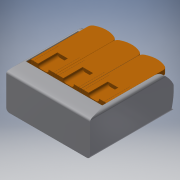
# Autodesk Inventor part: fc17-134
Saved by Autodesk Inventor 2017.1 (Build 211199000, 199)
## iProperties
Category: Electrical
Company: Autodesk Inc.
Created: 2016-12-21
Part Number: fc17-134
Catalog Web Link: https://eshop.wago.com/JPBC/0_5StartPage.jsp?supplierAID=221-413&catalogID=WAGO01&zone=7
Description: 221-413-COMPACT splicing connectors for all conductor types 3-conductor terminal block
Vendor: AndyMark Inc.
Document SubType Name: Modeling
Designer: Autodesk Inc.
Manufacturer: WAGO
Mass: 2.46 g
Surface Area: 17.0313 cm^2
Volume: 2.59959 cm^3
Density: 1 g/cm^3
Material: Generic
Appearance: PSOLRGB-175-175-175
Title: 221-413
Author: Autodesk Inc.
Comments: COMPACT splicing connectors for all conductor types 3-conductor terminal block
Keywords: FIRST Choice
Autodesk Inventor part; units mm, degrees
ref_plane "YZ Plane" through (0, 0, 0) normal (1, 0, 0) x (0, 1, 0)
ref_plane "XZ Plane" through (0, 0, 0) normal (0, 1, 0) x (-1, 0, 0)
ref_plane "XY Plane" through (0, 0, 0) normal (0, 0, 1) x (1, 0, 0)
sketch "Sketch_1" plane through (0, 0, 0) normal (0, 0, 1) x (1, 0, 0)
  line L0 (0, 7.2187) -> (0, 0)
  line L1 (0, 0) -> (18.4, 0)
  arc A0 (18.4, 0) -> (18.6, 0.2) centre (18.4, 0.2) ccw
  line L2 (18.6, 0.2) -> (18.6, 0.2905)
  arc A1 (18.6, 0.2905) -> (18.4845, 0.4717) centre (18.4, 0.2905) ccw
  line L3 (18.4845, 0.4717) -> (18.1022, 0.65)
  arc A2 (18.1022, 0.65) -> (18.5749, 4.9468) centre (4.69, 4.3) ccw
  arc A3 (18.5749, 4.9468) -> (18.4726, 5.3431) centre (17.576, 4.9002) ccw
  arc A4 (18.4726, 5.3431) -> (17.0892, 7.3213) centre (11.3, 1.8) ccw
  arc A5 (17.0892, 7.3213) -> (15.23, 8.15) centre (15.23, 5.65) ccw
  line L4 (15.23, 8.15) -> (3.62, 8.15)
  arc A6 (3.62, 8.15) -> (0.3643, 7.6999) centre (3.62, -3.85) ccw
  arc A7 (0.3643, 7.6999) -> (0, 7.2187) centre (0.5, 7.2187) ccw
  constraints: 16 point on circle, 10 end point, 8 centre point
extrude "Extrusion1" add sketch "Sketch_1" along normal blind 18.6
sketch "Sketch_5" plane through (0, 0, 0) normal (1, 0, 0) x (0, 1, 0)
  line L0 (9.15, 19.6) -> (-1, 19.6)
  line L1 (-1, 19.6) -> (-1, -1)
  line L2 (-1, -1) -> (9.15, -1)
  line L3 (9.15, -1) -> (9.15, 19.6)
  line L4 (7.45, 18.6) -> (0.7, 18.6)
  arc A0 (0.7, 18.6) -> (0, 17.9) centre (0.7, 17.9) ccw
  line L5 (0, 17.9) -> (0, 0.7)
  arc A1 (0, 0.7) -> (0.7, 0) centre (0.7, 0.7) ccw
  line L6 (0.7, 0) -> (7.45, 0)
  arc A2 (7.45, 0) -> (8.15, 0.7) centre (7.45, 0.7) ccw
  line L7 (8.15, 0.7) -> (8.15, 17.9)
  arc A3 (8.15, 17.9) -> (7.45, 18.6) centre (7.45, 17.9) ccw
  constraints: 16 end point, 8 point on circle, 4 centre point
extrude "Extrusion2" cut sketch "Sketch_5" along normal blind 18.6
sketch "Sketch_2" plane through (18.6, 0, 0) normal (1, 0, 0) x (0, 0, -1)
  line L0 (-6.15, 4.07) -> (-6.15, 1.35)
  arc A0 (-6.15, 1.35) -> (-5.45, 0.65) centre (-5.45, 1.35) ccw
  line L1 (-5.45, 0.65) -> (-1.95, 0.65)
  arc A1 (-1.95, 0.65) -> (-1.25, 1.35) centre (-1.95, 1.35) ccw
  line L2 (-1.25, 1.35) -> (-1.25, 4.07)
  arc A2 (-1.25, 4.07) -> (-1.95, 4.77) centre (-1.95, 4.07) ccw
  line L3 (-1.95, 4.77) -> (-5.45, 4.77)
  arc A3 (-5.45, 4.77) -> (-6.15, 4.07) centre (-5.45, 4.07) ccw
  constraints: 8 end point, 8 point on circle, 4 centre point
extrude "Extrusion3" cut sketch "Sketch_2" against normal blind 2
pattern_linear "Rectangular Pattern1" count 3 spacing 5.6 along (0, 0, 1) of "Extrusion3"
sketch "Sketch_4" plane through (18.6, 0, 0) normal (1, 0, 0) x (0, 0, -1)
  line L0 (-11.075, 7.3) -> (-11.075, 6.3)
  arc A0 (-11.075, 6.3) -> (-10.775, 6) centre (-10.775, 6.3) ccw
  line L1 (-10.775, 6) -> (-9.9408, 6)
  arc A1 (-9.9408, 6) -> (-8.6592, 6) centre (-9.3, 6.8) ccw
  line L2 (-8.6592, 6) -> (-7.825, 6)
  arc A2 (-7.825, 6) -> (-7.525, 6.3) centre (-7.825, 6.3) ccw
  line L3 (-7.525, 6.3) -> (-7.525, 7.3)
  arc A3 (-7.525, 7.3) -> (-7.825, 7.6) centre (-7.825, 7.3) ccw
  line L4 (-7.825, 7.6) -> (-8.6592, 7.6)
  arc A4 (-8.6592, 7.6) -> (-9.9408, 7.6) centre (-9.3, 6.8) ccw
  line L5 (-9.9408, 7.6) -> (-10.775, 7.6)
  arc A5 (-10.775, 7.6) -> (-11.075, 7.3) centre (-10.775, 7.3) ccw
  constraints: 12 end point, 12 point on circle, 6 centre point
extrude "Extrusion4" cut sketch "Sketch_4" against normal blind 2
sketch "Sketch_6" plane through (18.6, 0, 0) normal (1, 0, 0) x (0, 0, -1)
  line L0 (-6.5, 7) -> (-5.96, 7)
  line L1 (-5.96, 7) -> (-5.96, 8.15)
  line L2 (-5.96, 8.15) -> (-1.44, 8.15)
  line L3 (-1.44, 8.15) -> (-1.44, 7)
  line L4 (-1.44, 7) -> (-0.9, 7)
  line L5 (-0.9, 7) -> (-0.9, 9.15)
  line L6 (-0.9, 9.15) -> (-6.5, 9.15)
  line L7 (-6.5, 9.15) -> (-6.5, 7)
  constraints: 16 end point
extrude "Extrusion5" cut sketch "Sketch_6" against normal blind 14.98
pattern_linear "Rectangular Pattern2" count 2 spacing 11.2 along (0, 0, 1) of "Extrusion5"
sketch "Sketch_13" plane through (18.6, 0, 0) normal (1, 0, 0) x (0, 0, -1)
  line L0 (-12.1, 7) -> (-11.56, 7)
  line L1 (-11.56, 7) -> (-11.56, 8.15)
  line L2 (-11.56, 8.15) -> (-7.04, 8.15)
  line L3 (-7.04, 8.15) -> (-7.04, 7)
  line L4 (-7.04, 7) -> (-6.5, 7)
  line L5 (-6.5, 7) -> (-6.5, 9.15)
  line L6 (-6.5, 9.15) -> (-12.1, 9.15)
  line L7 (-12.1, 9.15) -> (-12.1, 7)
  constraints: 16 end point
extrude "Extrusion6" cut sketch "Sketch_13" against normal blind 14.98
sketch "Sketch_8" plane through (0, 8.15, 0) normal (0, 1, 0) x (1, 0, 0)
  line L0 (4.55, -5.98) -> (4.55, -6.48)
  line L1 (4.55, -6.48) -> (17.1821, -6.48)
  arc A0 (17.1821, -6.48) -> (18.0777, -5.925) centre (17.1821, -5.48) ccw
  arc A1 (18.0777, -5.925) -> (18.0777, -1.475) centre (13.6, -3.7) ccw
  arc A2 (18.0777, -1.475) -> (17.1821, -0.92) centre (17.1821, -1.92) ccw
  line L2 (17.1821, -0.92) -> (4.55, -0.92)
  line L3 (4.55, -0.92) -> (4.55, -1.42)
  line L4 (4.55, -1.42) -> (10.25, -1.42)
  arc A3 (10.65, -1.82) -> (10.25, -1.42) centre (10.25, -1.82) ccw
  line L5 (10.65, -1.82) -> (10.65, -5.58)
  arc A4 (10.25, -5.98) -> (10.65, -5.58) centre (10.25, -5.58) ccw
  line L6 (10.25, -5.98) -> (4.55, -5.98)
  constraints: 14 end point, 10 point on circle, 5 centre point
extrude "Extrusion7" add sketch "Sketch_8" against normal blind 1.1
pattern_linear "Rectangular Pattern3" count 3 spacing 5.6 along (0, 0, 1) of "Extrusion7"
sketch "Sketch_10" plane through (3.62, 0, 0) normal (1, 0, 0) x (0, 0, -1)
  arc A0 (-4.86, 8) -> (-4.26, 7.4) centre (-4.26, 8) ccw
  line L0 (-4.26, 7.4) -> (-3.14, 7.4)
  arc A1 (-3.14, 7.4) -> (-2.54, 8) centre (-3.14, 8) ccw
  line L1 (-2.54, 8) -> (-2.54, 8.15)
  line L2 (-2.54, 8.15) -> (-4.86, 8.15)
  line L3 (-4.86, 8.15) -> (-4.86, 8)
  constraints: 8 end point, 4 point on circle, 2 centre point
extrude "Extrusion8" cut sketch "Sketch_10" along normal blind 5.2
pattern_linear "Rectangular Pattern4" count 3 spacing 5.6 along (0, 0, 1) of "Extrusion8"
sketch "Sketch_12" plane through (0, 0, 0.9) normal (0, 0, 1) x (1, 0, 0)
  line L0 (3.62, 7) -> (4.55, 7)
  line L1 (4.55, 7) -> (4.55, 8.15)
  line L2 (4.55, 8.15) -> (3.62, 8.15)
  line L3 (3.62, 8.15) -> (3.62, 7)
  constraints: 8 end point
extrude "Extrusion9" cut sketch "Sketch_12" along normal blind 16.8
body "Solid1"
